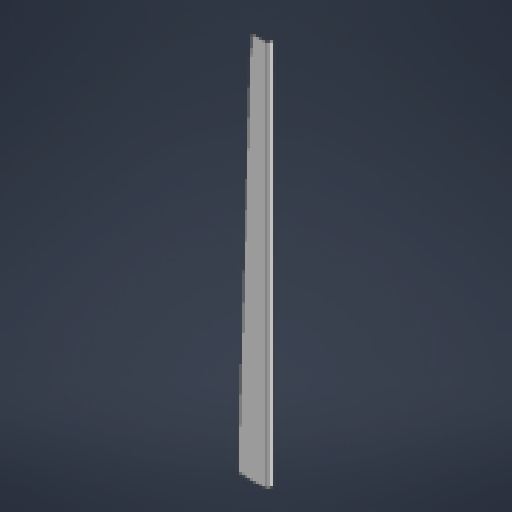
# Autodesk Inventor part: Part2_CPY
Saved by Autodesk Inventor 2026.2 (Build 302298000, 298)
## iProperties
Created: 2026-04-17
Part Number: Part2_CPY
Material: Generic
Document SubType Name: Sheet Metal
Designer: admin
Density: 1 g/cm^3
Sheet Metal Rule: Default
Appearance: Default
Author: admin
Autodesk Inventor part; units mm, degrees
ref_plane "YZ Plane" through (0, 0, 0) normal (1, 0, 0) x (0, 1, 0)
ref_plane "XZ Plane" through (0, 0, 0) normal (0, 1, 0) x (-1, 0, 0)
ref_plane "XY Plane" through (0, 0, 0) normal (0, 0, 1) x (1, 0, 0)
sketch "Sketch1" plane through (0, 0, 0) normal (0, 0, 1) x (1, 0, 0)
  line L0 (0, 0) -> (0, 1500)
  line L1 (0, 1500) -> (-136.5037, 1500)
  line L2 (-136.5037, 1500) -> (-162.6863, 0)
  line L3 (-162.6863, 0) -> (0, 0)
  line L4 (-137.3763, 1450.0076) -> (-142.3755, 1450.0949)
  line L5 (-142.3755, 1450.0949) -> (-167.687, 0)
  line L6 (-167.687, 0) -> (-162.6863, 0)
  line L7 (-167.687, 0) -> (-162.6863, 0) construction
  dimension "d0" = 1500
  dimension "d1" = 136.504
  dimension "d2" = 5
  dimension "d3" = 167.687
  dimension "d4" = 0
  dimension "d6" = 50
  dimension "d17" = 89
  measures "d0" distance of L0.start L0.end
  measures "d2" distance of L4.start L4.end
  measures "d4" distance of L5.end L6.start
  measures "d6" distance from line of L1.end L4
  measures "d17" angle of L3 L2
extrude "Plate1" add sketch "Sketch1" along normal blind 3.048
sketch "Sketch2" plane through (-3.048, 0, 3.048) normal (1, 0, 0) x (0, 1, 0)
  line L0 (1500, 0) -> (0, 0)
  line L1 (0, 0) -> (0, -25)
  line L2 (0, -25) -> (1500, -25)
  line L3 (1500, -25) -> (1500, 0)
  constraints: 6 end point, 1 horizontal, 1 perpendicular, 1 vertical
edge flange "Flange1" height 25 angle 90 thickness 3.048 bend radius 3.048 thickness toward (1, 0, 0) relief straight relief width 3.048 relief depth 1.524 edges at (0, 750, 0) wall of the first edge with corners at (-3.048, 1500, 3.048) (-3.048, 0, 3.048) (-3.048, 0, -21.952) (-3.048, 1500, -21.952)
bend "Bend1"
corner "Corner1"
equation "\"d5\" = Thickness"
equation "\"d7\" = BendReliefWidth"
equation "\"d8\" = BendReliefDepth"
equation "\"d9\" = MinimumRemnant"
equation "\"d10\" = TransitionRadius"
equation "\"d13\" = BendRadius"
equation "\"d14\" = CornerReliefSize"
equation "\"d15\" = GapSize"
equation "\"d16\" = JacobiRadiusSize"
equation "\"BendRadius\" = Thickness"
equation "\"BendReliefWidth\" = Thickness"
equation "\"BendReliefDepth\" = 0.5 * Thickness"
equation "\"CornerReliefSize\" = 4 * Thickness"
equation "\"MinimumRemnant\" = 2 * Thickness"
equation "\"TransitionRadius\" = BendRadius"
equation "\"JacobiRadiusSize\" = BendRadius"
equation "\"GapSize\" = Thickness"
equation "\"Thickness\" = 3.048"
body "Solid1"
